Autodesk Fusion 360 part; units mm, degrees
(part 5 of 5)
  spline S19 degree 5 poles (260.708, 93.7644) (260.6754, 93.7158) (260.6104, 93.6184) (260.5134, 93.4722) (260.385, 93.2769) (260.2261, 93.0322) (260.0688, 92.7871) (259.9132, 92.5414) (259.7592, 92.2951) (259.6068, 92.0484) (259.4561, 91.8011) (259.3071, 91.5533) (259.1598, 91.3051) (259.0141, 91.0563) (258.8702, 90.807) (258.728, 90.5573) (258.5875, 90.3071) (258.4488, 90.0564) (258.3118, 89.8052) (258.1766, 89.5536) (258.0432, 89.3016) (257.9116, 89.0491) (257.7819, 88.7961) (257.6539, 88.5428) (257.5278, 88.289) (257.4036, 88.0348) (257.2812, 87.7801) (257.1607, 87.5251) (257.0422, 87.2697) (256.9255, 87.0139) (256.8109, 86.7577) (256.6981, 86.5012) (256.5874, 86.2443) (256.4787, 85.987) (256.3721, 85.7294) (256.2675, 85.4715) (256.1649, 85.2132) (256.0644, 84.9546) (255.9661, 84.6956) (255.8699, 84.4364) (255.7758, 84.1769) (255.684, 83.9171) (255.5944, 83.657) (255.5072, 83.3966) (255.4222, 83.136) (255.3396, 82.8752) (255.2593, 82.6141) (255.1813, 82.3528) (255.1057, 82.0912) (255.0325, 81.8295) (254.9619, 81.5675) (254.8939, 81.3054) (254.8288, 81.0432) (254.7666, 80.7808) (254.7072, 80.5182) (254.6506, 80.2556) (254.5965, 79.9928) (254.5449, 79.7299) (254.4959, 79.467) (254.4499, 79.2039) (254.4074, 78.9409) (254.369, 78.6778) (254.3353, 78.4149) (254.3062, 78.1521) (254.2812, 77.8893) (254.2593, 77.6266) (254.2397, 77.364) (254.2223, 77.1015) (254.2078, 76.8391) (254.1989, 76.5772) (254.1992, 76.3159) (254.2099, 76.1077) (254.225, 75.952) (254.2386, 75.8484) (254.2461, 75.7967) knots -1 -1 -1 -1 -1 -1 -0.98571429 -0.97142857 -0.95714286 -0.94285714 -0.92857143 -0.91428571 -0.9 -0.88571429 -0.87142857 -0.85714286 -0.84285714 -0.82857143 -0.81428571 -0.8 -0.78571429 -0.77142857 -0.75714286 -0.74285714 -0.72857143 -0.71428571 -0.7 -0.68571429 -0.67142857 -0.65714286 -0.64285714 -0.62857143 -0.61428571 -0.6 -0.58571429 -0.57142857 -0.55714286 -0.54285714 -0.52857143 -0.51428571 -0.5 -0.48571429 -0.47142857 -0.45714286 -0.44285714 -0.42857143 -0.41428571 -0.4 -0.38571429 -0.37142857 -0.35714286 -0.34285714 -0.32857143 -0.31428571 -0.3 -0.28571429 -0.27142857 -0.25714286 -0.24285714 -0.22857143 -0.21428571 -0.2 -0.18571429 -0.17142857 -0.15714286 -0.14285714 -0.12857143 -0.11428571 -0.1 -0.08571429 -0.07142857 -0.05714286 -0.04285714 -0.02857143 -0.01428571 0 0 0 0 0 0
  line L19 (254.2461, 75.7967) -> (255.4273, 67.753)
  arc A39 (253.8013, 65.4937) -> (255.4273, 67.753) centre (253.4486, 67.4624) ccw
  arc A40 (253.8013, 65.4937) -> (243.7733, 62.8067) centre (264.6494, 4.9519) ccw
  arc A41 (241.2355, 63.9503) -> (243.7733, 62.8067) centre (243.0944, 64.688) ccw
  line L20 (241.2355, 63.9503) -> (238.2365, 71.5069)
  spline S20 degree 5 poles (238.2365, 71.5069) (238.2173, 71.5555) (238.1772, 71.6519) (238.1125, 71.7944) (238.0176, 71.9801) (237.8872, 72.2065) (237.7485, 72.4289) (237.6048, 72.6488) (237.4584, 72.8675) (237.3102, 73.0851) (237.1599, 73.3017) (237.0069, 73.5167) (236.8503, 73.7298) (236.6895, 73.9406) (236.5248, 74.1493) (236.3565, 74.3558) (236.1851, 74.5606) (236.0112, 74.7638) (235.8351, 74.9657) (235.6568, 75.1662) (235.4764, 75.3654) (235.2938, 75.563) (235.1087, 75.7592) (234.9212, 75.9538) (234.7313, 76.1468) (234.5391, 76.3383) (234.3449, 76.5284) (234.1486, 76.7171) (233.9504, 76.9044) (233.7503, 77.0903) (233.5483, 77.2749) (233.3445, 77.4582) (233.1387, 77.64) (232.9311, 77.8205) (232.7217, 77.9996) (232.5105, 78.1773) (232.2976, 78.3537) (232.0829, 78.5287) (231.8666, 78.7025) (231.6486, 78.8749) (231.4291, 79.046) (231.2079, 79.2157) (230.9851, 79.3842) (230.7608, 79.5513) (230.5349, 79.7171) (230.3075, 79.8816) (230.0786, 80.0449) (229.8482, 80.2068) (229.6164, 80.3674) (229.3831, 80.5267) (229.1484, 80.6847) (228.9123, 80.8415) (228.6748, 80.9969) (228.4359, 81.1511) (228.1957, 81.3039) (227.9542, 81.4555) (227.7113, 81.6058) (227.4671, 81.7548) (227.2216, 81.9026) (226.9748, 82.049) (226.7268, 82.1942) (226.4775, 82.3381) (226.227, 82.4807) (225.9753, 82.6221) (225.7223, 82.7622) (225.4682, 82.901) (225.2129, 83.0385) (224.9564, 83.1747) (224.6987, 83.3097) (224.44, 83.4434) (224.18, 83.5758) (223.9712, 83.6807) (223.814, 83.7588) (223.7091, 83.8107) (223.6565, 83.8365) knots 0 0 0 0 0 0 0.01428571 0.02857143 0.04285714 0.05714286 0.07142857 0.08571429 0.1 0.11428571 0.12857143 0.14285714 0.15714286 0.17142857 0.18571429 0.2 0.21428571 0.22857143 0.24285714 0.25714286 0.27142857 0.28571429 0.3 0.31428571 0.32857143 0.34285714 0.35714286 0.37142857 0.38571429 0.4 0.41428571 0.42857143 0.44285714 0.45714286 0.47142857 0.48571429 0.5 0.51428571 0.52857143 0.54285714 0.55714286 0.57142857 0.58571429 0.6 0.61428571 0.62857143 0.64285714 0.65714286 0.67142857 0.68571429 0.7 0.71428571 0.72857143 0.74285714 0.75714286 0.77142857 0.78571429 0.8 0.81428571 0.82857143 0.84285714 0.85714286 0.87142857 0.88571429 0.9 0.91428571 0.92857143 0.94285714 0.95714286 0.97142857 0.98571429 1 1 1 1 1 1
  arc A42 (223.6565, 83.8365) -> (216.8298, 79.8951) centre (264.6494, 4.9519) ccw
  spline S21 degree 5 poles (216.8298, 79.8951) (216.8259, 79.8367) (216.8183, 79.7198) (216.8074, 79.5447) (216.7938, 79.3114) (216.7785, 79.02) (216.7649, 78.7291) (216.753, 78.4385) (216.7427, 78.1482) (216.7342, 77.8584) (216.7273, 77.5689) (216.7221, 77.2798) (216.7187, 76.9911) (216.7169, 76.7028) (216.7169, 76.415) (216.7186, 76.1276) (216.7221, 75.8407) (216.7273, 75.5542) (216.7342, 75.2682) (216.743, 74.9827) (216.7535, 74.6977) (216.7657, 74.4133) (216.7798, 74.1293) (216.7957, 73.8459) (216.8134, 73.5631) (216.8329, 73.2808) (216.8542, 72.9991) (216.8774, 72.7181) (216.9024, 72.4376) (216.9293, 72.1577) (216.9581, 71.8785) (216.9887, 71.6) (217.0213, 71.3222) (217.0558, 71.045) (217.0923, 70.7686) (217.1306, 70.4929) (217.171, 70.2179) (217.2133, 69.9437) (217.2575, 69.6703) (217.3038, 69.3977) (217.3521, 69.1259) (217.4025, 68.855) (217.455, 68.585) (217.5096, 68.3159) (217.5664, 68.0477) (217.6252, 67.7805) (217.6862, 67.5143) (217.7494, 67.249) (217.8146, 66.9846) (217.8821, 66.7214) (217.9519, 66.4592) (218.0241, 66.1982) (218.0989, 65.9386) (218.1762, 65.6802) (218.256, 65.4232) (218.3383, 65.1674) (218.4228, 64.9128) (218.5096, 64.6593) (218.5987, 64.4071) (218.6903, 64.1562) (218.785, 63.9072) (218.8833, 63.6602) (218.9856, 63.4156) (219.0918, 63.1734) (219.2015, 62.9334) (219.3139, 62.695) (219.4283, 62.4578) (219.5444, 62.2217) (219.6631, 61.9873) (219.7863, 61.756) (219.9172, 61.5298) (220.0306, 61.3548) (220.1216, 61.2276) (220.1851, 61.1446) (220.2175, 61.1036) knots -1 -1 -1 -1 -1 -1 -0.98571429 -0.97142857 -0.95714286 -0.94285714 -0.92857143 -0.91428571 -0.9 -0.88571429 -0.87142857 -0.85714286 -0.84285714 -0.82857143 -0.81428571 -0.8 -0.78571429 -0.77142857 -0.75714286 -0.74285714 -0.72857143 -0.71428571 -0.7 -0.68571429 -0.67142857 -0.65714286 -0.64285714 -0.62857143 -0.61428571 -0.6 -0.58571429 -0.57142857 -0.55714286 -0.54285714 -0.52857143 -0.51428571 -0.5 -0.48571429 -0.47142857 -0.45714286 -0.44285714 -0.42857143 -0.41428571 -0.4 -0.38571429 -0.37142857 -0.35714286 -0.34285714 -0.32857143 -0.31428571 -0.3 -0.28571429 -0.27142857 -0.25714286 -0.24285714 -0.22857143 -0.21428571 -0.2 -0.18571429 -0.17142857 -0.15714286 -0.14285714 -0.12857143 -0.11428571 -0.1 -0.08571429 -0.07142857 -0.05714286 -0.04285714 -0.02857143 -0.01428571 0 0 0 0 0 0
  line L21 (220.2175, 61.1036) -> (225.2623, 54.7282)
  arc A43 (224.9837, 51.9586) -> (225.2623, 54.7282) centre (223.6939, 53.4871) ccw
  arc A44 (224.9837, 51.9586) -> (217.6427, 44.6176) centre (264.6494, 4.9519) ccw
  arc A45 (214.8731, 44.339) -> (217.6427, 44.6176) centre (216.1142, 45.9074) ccw
  line L22 (214.8731, 44.339) -> (208.4977, 49.3838)
  spline S22 degree 5 poles (208.4977, 49.3838) (208.4567, 49.4162) (208.3737, 49.4797) (208.2465, 49.5707) (208.0715, 49.6841) (207.8453, 49.815) (207.614, 49.9382) (207.3796, 50.0569) (207.1435, 50.173) (206.9063, 50.2874) (206.6679, 50.3998) (206.4278, 50.5095) (206.1857, 50.6157) (205.9411, 50.718) (205.6941, 50.8163) (205.4451, 50.911) (205.1942, 51.0026) (204.942, 51.0917) (204.6885, 51.1784) (204.4339, 51.263) (204.1781, 51.3453) (203.9211, 51.4251) (203.6627, 51.5024) (203.4031, 51.5772) (203.1421, 51.6494) (202.8799, 51.7192) (202.6167, 51.7867) (202.3523, 51.8519) (202.087, 51.9151) (201.8208, 51.9761) (201.5536, 52.0349) (201.2854, 52.0917) (201.0163, 52.1463) (200.7463, 52.1988) (200.4754, 52.2492) (200.2036, 52.2975) (199.931, 52.3438) (199.6576, 52.388) (199.3834, 52.4303) (199.1084, 52.4707) (198.8327, 52.509) (198.5563, 52.5455) (198.2791, 52.58) (198.0013, 52.6125) (197.7227, 52.6432) (197.4436, 52.672) (197.1637, 52.6989) (196.8832, 52.7239) (196.6022, 52.7471) (196.3205, 52.7684) (196.0382, 52.7879) (195.7554, 52.8056) (195.472, 52.8215) (195.188, 52.8356) (194.9035, 52.8478) (194.6186, 52.8583) (194.3331, 52.8671) (194.0471, 52.874) (193.7606, 52.8792) (193.4737, 52.8827) (193.1863, 52.8844) (192.8985, 52.8844) (192.6102, 52.8826) (192.3215, 52.8792) (192.0324, 52.874) (191.7429, 52.8671) (191.4531, 52.8586) (191.1628, 52.8483) (190.8722, 52.8364) (190.5813, 52.8228) (190.2899, 52.8075) (190.0566, 52.7939) (189.8815, 52.783) (189.7646, 52.7754) (189.7062, 52.7715) knots 0 0 0 0 0 0 0.01428571 0.02857143 0.04285714 0.05714286 0.07142857 0.08571429 0.1 0.11428571 0.12857143 0.14285714 0.15714286 0.17142857 0.18571429 0.2 0.21428571 0.22857143 0.24285714 0.25714286 0.27142857 0.28571429 0.3 0.31428571 0.32857143 0.34285714 0.35714286 0.37142857 0.38571429 0.4 0.41428571 0.42857143 0.44285714 0.45714286 0.47142857 0.48571429 0.5 0.51428571 0.52857143 0.54285714 0.55714286 0.57142857 0.58571429 0.6 0.61428571 0.62857143 0.64285714 0.65714286 0.67142857 0.68571429 0.7 0.71428571 0.72857143 0.74285714 0.75714286 0.77142857 0.78571429 0.8 0.81428571 0.82857143 0.84285714 0.85714286 0.87142857 0.88571429 0.9 0.91428571 0.92857143 0.94285714 0.95714286 0.97142857 0.98571429 1 1 1 1 1 1
  arc A46 (189.7062, 52.7715) -> (185.7648, 45.9448) centre (264.6494, 4.9519) ccw
  spline S23 degree 5 poles (185.7648, 45.9448) (185.7906, 45.8922) (185.8425, 45.7872) (185.9206, 45.6301) (186.0255, 45.4213) (186.1579, 45.1613) (186.2916, 44.9025) (186.4266, 44.6449) (186.5628, 44.3884) (186.7003, 44.1331) (186.8391, 43.879) (186.9792, 43.626) (187.1206, 43.3743) (187.2632, 43.1238) (187.4071, 42.8745) (187.5523, 42.6265) (187.6987, 42.3797) (187.8465, 42.1342) (187.9955, 41.89) (188.1458, 41.6471) (188.2974, 41.4056) (188.4502, 41.1654) (188.6044, 40.9265) (188.7598, 40.689) (188.9166, 40.4529) (189.0746, 40.2182) (189.2339, 39.9849) (189.3945, 39.7531) (189.5564, 39.5227) (189.7197, 39.2938) (189.8842, 39.0664) (190.05, 38.8405) (190.2171, 38.6162) (190.3856, 38.3934) (190.5553, 38.1722) (190.7264, 37.9527) (190.8988, 37.7347) (191.0726, 37.5184) (191.2476, 37.3037) (191.424, 37.0908) (191.6017, 36.8796) (191.7808, 36.6702) (191.9613, 36.4626) (192.1431, 36.2568) (192.3264, 36.053) (192.511, 35.851) (192.6969, 35.6509) (192.8842, 35.4527) (193.0729, 35.2564) (193.263, 35.0622) (193.4545, 34.87) (193.6475, 34.6801) (193.8421, 34.4926) (194.0383, 34.3075) (194.2359, 34.1249) (194.4351, 33.9445) (194.6356, 33.7662) (194.8375, 33.5901) (195.0407, 33.4162) (195.2455, 33.2448) (195.452, 33.0765) (195.6607, 32.9117) (195.8715, 32.751) (196.0846, 32.5944) (196.2996, 32.4414) (196.5162, 32.2911) (196.7338, 32.1429) (196.9524, 31.9965) (197.1724, 31.8528) (197.3948, 31.7141) (197.6212, 31.5837) (197.8069, 31.4888) (197.9494, 31.4241) (198.0458, 31.384) (198.0944, 31.3648) knots -1 -1 -1 -1 -1 -1 -0.98571429 -0.97142857 -0.95714286 -0.94285714 -0.92857143 -0.91428571 -0.9 -0.88571429 -0.87142857 -0.85714286 -0.84285714 -0.82857143 -0.81428571 -0.8 -0.78571429 -0.77142857 -0.75714286 -0.74285714 -0.72857143 -0.71428571 -0.7 -0.68571429 -0.67142857 -0.65714286 -0.64285714 -0.62857143 -0.61428571 -0.6 -0.58571429 -0.57142857 -0.55714286 -0.54285714 -0.52857143 -0.51428571 -0.5 -0.48571429 -0.47142857 -0.45714286 -0.44285714 -0.42857143 -0.41428571 -0.4 -0.38571429 -0.37142857 -0.35714286 -0.34285714 -0.32857143 -0.31428571 -0.3 -0.28571429 -0.27142857 -0.25714286 -0.24285714 -0.22857143 -0.21428571 -0.2 -0.18571429 -0.17142857 -0.15714286 -0.14285714 -0.12857143 -0.11428571 -0.1 -0.08571429 -0.07142857 -0.05714286 -0.04285714 -0.02857143 -0.01428571 0 0 0 0 0 0
  line L23 (198.0944, 31.3648) -> (205.651, 28.3658)
  arc A47 (206.7946, 25.828) -> (205.651, 28.3658) centre (204.9133, 26.5069) ccw
  circle A48 centre (264.6494, 4.9519) radius 5
  circle A49 centre (264.6494, 4.9519) radius 5
  dimension "d43" = 10
  constraint concentric A0 A49
  measures "d43" diameter of A49
extrude "Extrude3'" add sketch "Sketch1" along normal blind 20 and the other way blind 32.17 contours A97 A98 sketch seen with x (1, 0, 0) y (0, 1, 0) z (0, 0, 1) at (264.6494, 4.9519, 0) bodies 2 in component "Spur Gear 12 teeth"
copy_body "Body->Comp1" bodies 1 removing the originals makes body 3 in component "Component"
copy_body "Body->Comp1'" bodies 2 removing the originals makes body 4 in component "Component'"
component "Spur Gear 24 teeth" placed x (1, 0, 0) y (0, 1, 0) z (0, 0, 1) at (0, 0, -20)
component "Spur Gear 12 teeth" placed x (1, 0, 0) y (0, 1, 0) z (0, 0, 1) at (-264.6494, -4.9519, -20)
component "Component" placed x (1, 0, 0) y (0, 1, 0) z (0, 0, 1) at (0, 0, 0) in component "Spur Gear 24 teeth"
component "Component'" placed x (1, 0, 0) y (0, 1, 0) z (0, 0, 1) at (0, 0, 0) in component "Spur Gear 12 teeth"
